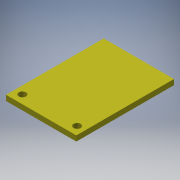
# Autodesk Inventor part: ADXL_345
Saved by Autodesk Inventor 2016 SP1 (Build 200210100, 210)
## iProperties
Created: 2016-02-02
Part Number: ADXL_345
Material: ABS Plastic
Document SubType Name: Modeling
Designer: steele
Density: 1.06 g/cm^3
Appearance: Canary
Author: steele
Autodesk Inventor part; units mm, degrees
ref_plane "XZ Plane" through (0, 0, 0) normal (0, 1, 0) x (-1, 0, 0)
sketch "Sketch1" plane through (0, 0, 0) normal (0, 1, 0) x (-1, 0, 0)
  line L0 (11.43, 15.875) -> (-11.43, 15.875)
  line L1 (-11.43, 15.875) -> (-11.43, -15.875)
  line L2 (-11.43, -15.875) -> (11.43, -15.875)
  line L3 (11.43, -15.875) -> (11.43, 15.875)
  line L4 (11.43, 15.875) -> (-11.43, -15.875) construction
  line L5 (-11.43, 15.875) -> (11.43, -15.875) construction
  point P0 (0, 0)
  dimension "d0" = 22.86
  dimension "d1" = 31.75
  constraints: 12 end point, 2 midpoint, 2 parallel, 1 horizontal, 1 perpendicular
  measures "d0" distance of L0.start L0.end
  measures "d1" distance of L2.end L0.start
extrude "Extrusion1" add sketch "Sketch1" along normal blind 1.7272
sketch "Sketch2" plane through (0, 1.7272, 0) normal (0, 1, 0) x (1, 0, 0)
  line L0 (-11.2735, -13.081) -> (11.43, -13.081) construction
  line L1 (11.43, -15.875) -> (11.43, 15.875) construction
  circle A0 centre (-8.89, -13.081) radius 1.1684
  circle A1 centre (8.89, -13.081) radius 1.1684
  line L2 (-11.43, -15.875) -> (11.43, -15.875) projected
  line L3 (-11.43, 15.875) -> (-11.43, -15.875) projected
  point P0 (0, 0)
  dimension "d4" = 2.794
  dimension "d5" = 2.54
  dimension "d6" = 2.54
  dimension "d7" = 2.3368
  dimension "d8" = 2.3368
  constraints: 3 point on line, 2 centre point, 2 end point, 1 horizontal
  measures "d4" distance between parallel lines of L0 L2
  measures "d5" distance from line of A0.centre L3
  measures "d6" distance from line of L1 A1.centre
  measures "d7" diameter of A0
  measures "d8" diameter of A1
extrude "Extrusion2" cut sketch "Sketch2" against normal through all
equation "\"d0\" = boardWidth"
equation "\"d1\" = boardLength"
equation "\"d2\" = boardThickness"
equation "\"d4\" = centerLineForHoles"
equation "\"d5\" = holeDistanceFromEdge"
equation "\"d6\" = holeDistanceFromEdge"
equation "\"d7\" = holeDiam"
equation "\"d8\" = holeDiam"
equation "\"d9\" = boardThickness"
equation "\"boardWidth\" = 22.86"
equation "\"boardLength\" = 31.75"
equation "\"boardThickness\" = 1.7272"
equation "\"componentHeightAboveBoard\" = 3.9878"
equation "\"headerHeightAboveBard\" = 8.7376"
equation "\"holeDiam\" = 2.3368"
equation "\"centerLineForHoles\" = 2.794"
equation "\"holeDistanceFromEdge\" = 2.54"
equation "\"supportWidth\" = 25.4"
body "Solid1"
